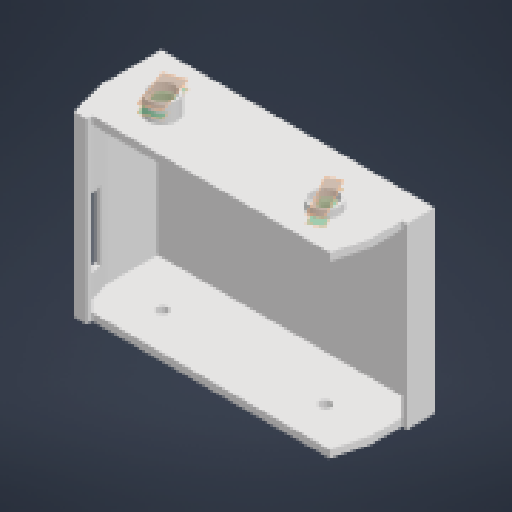
# Autodesk Inventor part: body
Saved by Autodesk Inventor 2025 (Build 290162000, 162)
## iProperties
Created: 2024-12-26
Part Number: body
Material: Типовые
Document SubType Name: Modeling
Designer: khrip
Density: 1 g/cm^3
Appearance: По умолчанию
Author: khrip
Autodesk Inventor part; units mm, degrees
ref_plane "РабПлоскость1" through (0, 0, 10) normal (0, 0, 1) x (1, 0, 0)
sketch "Эскиз1" plane through (0, 0, 10) normal (0, 0, 1) x (1, 0, 0)
  line L0 (-107.5, 70) -> (107.5, 70)
  line L1 (107.5, 70) -> (107.5, -70)
  line L2 (107.5, -70) -> (-107.5, -70)
  line L3 (-107.5, -70) -> (-107.5, 70)
  line L4 (-107.5, 70) -> (107.5, -70) construction
  line L5 (107.5, 70) -> (-107.5, -70) construction
  point P0 (0, 0)
  dimension "d1" = 215
  dimension "d2" = 140
  constraints: 12 end point, 2 midpoint, 2 parallel, 1 horizontal, 1 perpendicular
  measures "d1" distance of L1.end L2.end
  measures "d2" distance of L0.end L1.end
extrude "Выдавливание1" add sketch "Эскиз1" along normal blind 7
sketch "Эскиз2" plane through (-107.5, 70, 10) normal (0, 1, 0) x (1, 0, 0)
  line L0 (215, 0) -> (0, 0) projected
  line L1 (0, 0) -> (0, -7) projected
  line L2 (215, -7) -> (0, -7) projected
  line L3 (215, 0) -> (215, -7) projected
  line L4 (154.9795, -76.2499) -> (152.5795, -76.2499) projected
  line L5 (155.2294, -76) -> (154.9795, -76.2499) projected
  line L6 (159.8295, -76) -> (155.2294, -76) projected
  line L7 (160.0795, -76.2499) -> (159.8295, -76) projected
  line L8 (162.4795, -76.2499) -> (160.0795, -76.2499) projected
  line L9 (162.7294, -76) -> (162.4795, -76.2499) projected
  line L10 (167.3295, -76) -> (162.7294, -76) projected
  line L11 (167.5795, -76.2499) -> (167.3295, -76) projected
  line L12 (169.9795, -76.2499) -> (167.5795, -76.2499) projected
  line L13 (170.2294, -76) -> (169.9795, -76.2499) projected
  line L14 (174.8295, -76) -> (170.2294, -76) projected
  line L15 (175.0795, -76.2499) -> (174.8295, -76) projected
  line L16 (177.4795, -76.2499) -> (175.0795, -76.2499) projected
  line L17 (177.7294, -76) -> (177.4795, -76.2499) projected
  line L18 (182.3295, -76) -> (177.7294, -76) projected
  line L19 (182.5795, -76.2499) -> (182.3295, -76) projected
  line L20 (184.9795, -76.2499) -> (182.5795, -76.2499) projected
  line L21 (185.2294, -76) -> (184.9795, -76.2499) projected
  line L22 (189.8295, -76) -> (185.2294, -76) projected
  line L23 (190.0795, -76.2499) -> (189.8295, -76) projected
  line L24 (192.4795, -76.2499) -> (190.0795, -76.2499) projected
  line L25 (192.7294, -76) -> (192.4795, -76.2499) projected
  line L26 (197.3295, -76) -> (192.7294, -76) projected
  line L27 (197.5795, -76.2499) -> (197.3295, -76) projected
  line L28 (199.9795, -76.2499) -> (197.5795, -76.2499) projected
  line L29 (200.2294, -76) -> (199.9795, -76.2499) projected
  line L30 (204.8295, -76) -> (200.2294, -76) projected
  line L31 (205.0795, -76.2499) -> (204.8295, -76) projected
  line L32 (207.4152, -76.2499) -> (205.0795, -76.2499) projected
  arc A0 (208.0813, -72.8208) -> (207.4152, -76.2499) centre (232.2295, -79.2913) ccw projected
  line L33 (208.0813, -72.8208) -> (215, -47) projected
  line L34 (215, -22) -> (215, -47) projected
  line L35 (215, -22) -> (211, -22) projected
  line L36 (211, -22) -> (211, -46.4734) projected
  line L37 (211, -46.4734) -> (204.1602, -72) projected
  line L38 (204.1602, -72) -> (150.3397, -72) projected
  line L39 (150.3397, -72) -> (150.3397, -76) projected
  line L40 (152.3295, -76) -> (150.3397, -76) projected
  line L41 (152.5795, -76.2499) -> (152.3295, -76) projected
  line L42 (107.5, 0) -> (107.5, -94.8503)
  line L43 (15.0205, -76.2499) -> (17.4205, -76.2499)
  line L44 (7.5848, -76.2499) -> (9.9205, -76.2499)
  arc A1 (7.5848, -76.2499) -> (6.9187, -72.8208) centre (-17.2295, -79.2913) ccw
  line L45 (6.9187, -72.8208) -> (0, -47)
  line L46 (0, -22) -> (0, -47)
  line L47 (0, -22) -> (4, -22)
  line L48 (4, -22) -> (4, -46.4734)
  line L49 (4, -46.4734) -> (10.8398, -72)
  line L50 (10.8398, -72) -> (64.6603, -72)
  line L51 (215, -22) -> (211, -22)
  line L52 (211, -22) -> (211, -7)
  line L53 (211, -7) -> (215, -7)
  line L54 (215, -7) -> (215, -22)
  line L55 (4, -22) -> (0, -22)
  line L56 (0, -22) -> (0, -7)
  line L57 (0, -7) -> (4, -7)
  line L58 (4, -7) -> (4, -22)
  line L59 (17.8835, -76.2499) -> (7.5848, -76.2499)
  line L60 (10.8398, -72) -> (17.8835, -72)
  line L61 (17.8835, -72) -> (17.8835, -76.2499)
  point P0 (107.5, 10)
  point P1 (17.8835, -72)
  constraints: 40 end point, 12 symmetric about line, 5 parallel, 3 horizontal, 2 perpendicular, 2 point on circle, 1 centre point, 1 midpoint, 1 point on line, 1 vertical, 1 other
extrude "Выдавливание2" add sketch "Эскиз2" against normal up to surface (140 mm away) contours L54 L35 L52 L2 | L2 L58 L47 L56 | L47 L48 L49 L50 L61 L59 L43 L44 A1 L45 L46
sketch "Эскиз3" plane through (-107.5, -70, 10) normal (0, -1, 0) x (1, 0, 0)
  line L0 (0, 0) -> (215, 0) projected
  line L1 (215, 0) -> (215, 22) projected
  line L2 (211, 22) -> (215, 22) projected
  line L3 (211, 7) -> (211, 22) projected
  line L4 (4, 7) -> (211, 7) projected
  line L5 (4, 46.4734) -> (4, 7) projected
  line L6 (10.8398, 72) -> (4, 46.4734) projected
  line L7 (17.8835, 72) -> (10.8398, 72) projected
  line L8 (17.8835, 76.2499) -> (17.8835, 72) projected
  line L9 (7.5848, 76.2499) -> (17.8835, 76.2499) projected
  arc A0 (6.9187, 72.8208) -> (7.5848, 76.2499) centre (-17.2295, 79.2913) ccw projected
  line L10 (0, 47) -> (6.9187, 72.8208) projected
  line L11 (0, 0) -> (0, 47) projected
  line L12 (205.0795, 76.2499) -> (207.4152, 76.2499) projected
  line L13 (204.8295, 76) -> (205.0795, 76.2499) projected
  line L14 (200.2294, 76) -> (204.8295, 76) projected
  line L15 (199.9795, 76.2499) -> (200.2294, 76) projected
  line L16 (197.5795, 76.2499) -> (199.9795, 76.2499) projected
  line L17 (197.3295, 76) -> (197.5795, 76.2499) projected
  line L18 (192.7294, 76) -> (197.3295, 76) projected
  line L19 (192.4795, 76.2499) -> (192.7294, 76) projected
  line L20 (190.0795, 76.2499) -> (192.4795, 76.2499) projected
  line L21 (189.8295, 76) -> (190.0795, 76.2499) projected
  line L22 (185.2294, 76) -> (189.8295, 76) projected
  line L23 (184.9795, 76.2499) -> (185.2294, 76) projected
  line L24 (182.5795, 76.2499) -> (184.9795, 76.2499) projected
  line L25 (182.3295, 76) -> (182.5795, 76.2499) projected
  line L26 (177.7294, 76) -> (182.3295, 76) projected
  line L27 (177.4795, 76.2499) -> (177.7294, 76) projected
  line L28 (175.0795, 76.2499) -> (177.4795, 76.2499) projected
  line L29 (174.8295, 76) -> (175.0795, 76.2499) projected
  line L30 (170.2294, 76) -> (174.8295, 76) projected
  line L31 (169.9795, 76.2499) -> (170.2294, 76) projected
  line L32 (167.5795, 76.2499) -> (169.9795, 76.2499) projected
  line L33 (167.3295, 76) -> (167.5795, 76.2499) projected
  line L34 (162.7294, 76) -> (167.3295, 76) projected
  line L35 (162.4795, 76.2499) -> (162.7294, 76) projected
  line L36 (160.0795, 76.2499) -> (162.4795, 76.2499) projected
  line L37 (159.8295, 76) -> (160.0795, 76.2499) projected
  line L38 (155.2294, 76) -> (159.8295, 76) projected
  line L39 (154.9795, 76.2499) -> (155.2294, 76) projected
  line L40 (152.5795, 76.2499) -> (154.9795, 76.2499) projected
  line L41 (152.3295, 76) -> (152.5795, 76.2499) projected
  line L42 (150.3397, 76) -> (152.3295, 76) projected
  line L43 (150.3397, 72) -> (150.3397, 76) projected
  line L44 (150.3397, 72) -> (204.1602, 72) projected
  line L45 (204.1602, 72) -> (211, 46.4734) projected
  line L46 (211, 46.4734) -> (211, 22) projected
  line L47 (211, 22) -> (215, 22) projected
  line L48 (215, 22) -> (215, 47) projected
  line L49 (215, 47) -> (208.0813, 72.8208) projected
  arc A1 (207.4152, 76.2499) -> (208.0813, 72.8208) centre (232.2295, 79.2913) ccw projected
  line L50 (17.8835, 76.2499) -> (207.9879, 76)
  line L51 (17.8835, 72) -> (150.3397, 72)
  circle A2 centre (43.62, 42.82) radius 4 projected
  circle A3 centre (171.38, 42.82) radius 4.3 projected
  point P0 (107.5, -10)
  constraints: 4 end point, 1 collinear
extrude "Выдавливание3" add sketch "Эскиз3" against normal blind 6 contours L3 L4 L5 L6 L7 L51 L44 L45 L46
sketch "Эскиз4" plane through (-107.5, -70, 10) normal (0, -1, 0) x (1, 0, 0)
  circle A0 centre (43.62, 42.82) radius 9.5 projected
  circle A1 centre (43.62, 42.82) radius 11.5
  point P0 (107.5, -10)
  dimension "d9" = 23
  constraints: 1 centre point, 1 coincident
  measures "d9" diameter of A1
ref_plane "РабПлоскость2" through (-75.6513, -84.5, 41.0487) normal (0, -1, 0) x (0.941, 0, -0.3385)
extrude "Выдавливание4" add sketch "Эскиз4" along normal up to surface (14.5 mm away)
sketch "Эскиз5" plane through (-63.88, -70, 52.82) normal (0, -1, 0) x (1, 0, 0)
  circle A0 centre (0, 0) radius 7.707 projected
  circle A1 centre (0, 0) radius 9.5 projected
  point P0 (63.88, -52.82)
ref_plane "РабПлоскость3" through (-75.6513, -78.5, 41.0487) normal (0, 1, 0) x (0.3385, 0, 0.941)
extrude "Выдавливание5" add sketch "Эскиз5" along normal up to surface (8.5 mm away)
sketch "Эскиз6" plane through (-107.5, -70, 10) normal (0, -1, 0) x (1, 0, 0)
  point P0 (107.5, -10)
sketch "Эскиз7" plane through (-107.5, -70, 10) normal (0, -1, 0) x (1, 0, 0)
  circle A0 centre (171.38, 42.82) radius 7.707 projected
  circle A1 centre (171.38, 42.82) radius 9.5 projected
  point P0 (107.5, -10)
ref_plane "РабПлоскость4" through (51.3812, -70.5, 40.3212) normal (0, 1, 0) x (0.4829, 0, 0.8757)
extrude "Выдавливание6" add sketch "Эскиз7" along normal up to surface (0.5 mm away)
sketch "Эскиз8" plane through (-107.5, -70, 10) normal (0, -1, 0) x (1, 0, 0)
  circle A0 centre (171.38, 42.82) radius 9.5 projected
  circle A1 centre (171.38, 42.82) radius 11.5
  point P0 (107.5, -10)
  dimension "d16" = 23
  constraints: 1 centre point, 1 coincident
  measures "d16" diameter of A1
ref_plane "РабПлоскость5" through (51.3812, -76.5, 40.3212) normal (0, -1, 0) x (0.8757, 0, -0.4829)
extrude "Выдавливание7" add sketch "Эскиз8" along normal up to surface (6.5 mm away)
mirror "Зеркальное отражение1" about plane through (0, 0, 0) normal (0, 1, 0) of "Выдавливание3", "Выдавливание4", "Выдавливание5", "Выдавливание6", "Выдавливание7"
sketch "Эскиз9" plane through (-107.5, -70, 10) normal (-1, 0, 0) x (0, 0, 1)
  line L0 (69.9727, 77.7173) -> (54.1331, 77.7173)
  line L1 (54.1331, 77.7173) -> (54.1331, 23.438)
  line L2 (54.1331, 23.438) -> (69.9727, 23.438)
  line L3 (69.9727, 23.438) -> (69.9727, 77.7173)
  point P0 (-10, 70)
  constraints: 8 end point, 2 parallel, 1 horizontal, 1 perpendicular
extrude "Выдавливание8" cut sketch "Эскиз9" against normal blind 10
ref_plane "РабПлоскость6" through (-75.6513, 84.5, 41.0487) normal (0, -1, 0) x (0.941, 0, -0.3385)
ref_plane "РабПлоскость7" through (-75.6513, 78.5, 41.0487) normal (0, 1, 0) x (0.3385, 0, 0.941)
ref_plane "РабПлоскость8" through (51.3812, 70.5, 40.3212) normal (0, 1, 0) x (0.4829, 0, 0.8757)
ref_plane "РабПлоскость9" through (51.3812, 76.5, 40.3212) normal (0, -1, 0) x (0.8757, 0, -0.4829)
